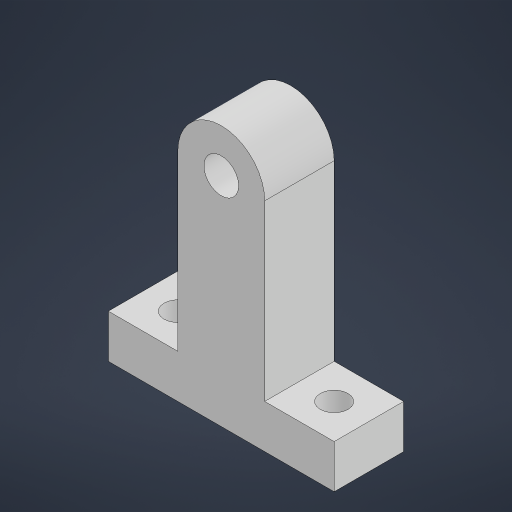
# Autodesk Inventor part: Mount_left
Saved by Autodesk Inventor 2024.2 (Build 282272000, 272)
## iProperties
Created: 2024-02-18
Part Number: Mount_left
Material: 一般
Document SubType Name: Modeling
Designer: Hanaoka
Density: 1 g/cm^3
Appearance: 既定
Author: Hanaoka
Autodesk Inventor part; units mm, degrees
ref_plane "YZ Plane" through (0, 0, 0) normal (1, 0, 0) x (0, 1, 0)
ref_plane "XZ Plane" through (0, 0, 0) normal (0, 1, 0) x (-1, 0, 0)
ref_plane "XY Plane" through (0, 0, 0) normal (0, 0, 1) x (1, 0, 0)
sketch "スケッチ1" plane through (0, 0, 0) normal (0, 0, 1) x (1, 0, 0)
  line L0 (0, 0) -> (0, 2.5)
  line L1 (0, 2.5) -> (4, 2.5)
  line L2 (0, 0) -> (13, 0)
  line L3 (13, 0) -> (13, 2.5)
  line L4 (13, 2.5) -> (9, 2.5)
  line L5 (9, 2.5) -> (9, 12.5)
  line L6 (4, 2.5) -> (4, 12.5)
  arc A0 (9, 12.5) -> (4, 12.5) centre (6.5, 12.5) ccw
  circle A1 centre (6.5, 12.5) radius 1
  dimension "d1" = 2.5
  dimension "d3" = 4
  dimension "d14" = 5
  dimension "d15" = 2
  dimension "d19" = 10
  constraints: 14 end point, 3 vertical, 2 centre point, 2 equal length, 2 perpendicular, 2 point on circle, 2 point on line, 1 coincident, 1 horizontal, 1 tangent
  measures "d1" distance of L2.end L3.end
  measures "d3" distance of L0.end L1.end
  measures "d14" distance of L1.end L4.end
  measures "d15" diameter of A1
  measures "d19" distance of L1.end L6.end
extrude "押し出し1" add sketch "スケッチ1" along normal blind 4
sketch "スケッチ2" plane through (0, 0, 0) normal (0, -1, 0) x (1, 0, 0)
  line L0 (13, 0) -> (9, 0) projected
  line L1 (9, 0) -> (9, 4) projected
  line L2 (13, 4) -> (9, 4) projected
  line L3 (13, 0) -> (13, 4) projected
  line L4 (4, 0) -> (0, 0) projected
  line L5 (0, 0) -> (0, 4) projected
  line L6 (4, 4) -> (0, 4) projected
  line L7 (4, 0) -> (4, 4) projected
  line L8 (4, 0) -> (0, 4) construction
  line L9 (4, 4) -> (0, 0) construction
  line L10 (9, 4) -> (13, 0) construction
  line L11 (13, 4) -> (9, 0) construction
  circle A0 centre (11, 2) radius 0.8
  circle A1 centre (2, 2) radius 0.8
  dimension "d10" = 1.6
  constraints: 8 end point, 2 centre point, 2 midpoint, 2 perpendicular, 1 equal radius
  measures "d10" diameter of A0
extrude "押し出し2" cut sketch "スケッチ2" against normal up to surface (2.5 mm away) contours A0 | A1
